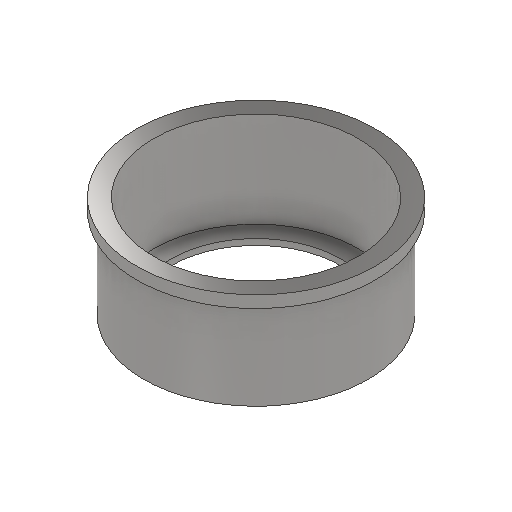
# Autodesk Inventor part: B_pipe_flange_spacer_5
Saved by Autodesk Inventor 2026.2 (Build 302298000, 298)
## iProperties
Created: 2026-07-10
Part Number: B_pipe_flange_spacer_5
Material: ステンレス鋼
Document SubType Name: Modeling
Designer: zetsu
Density: 8 g/cm^3
Appearance: 半つや出し
Author: zetsu
Autodesk Inventor part; units mm, degrees
ref_plane "YZ Plane" through (0, 0, 0) normal (1, 0, 0) x (0, 1, 0)
ref_plane "XZ Plane" through (0, 0, 0) normal (0, 1, 0) x (-1, 0, 0)
ref_plane "XY Plane" through (0, 0, 0) normal (0, 0, 1) x (1, 0, 0)
sketch "スケッチ1" plane through (0, 0, 0) normal (0, 1, 0) x (-1, 0, 0)
  circle A0 centre (0, 0) radius 18.85
  circle A1 centre (0, 0) radius 14.2
  dimension "d0" = 37.7
  dimension "d1" = 28.4
  constraints: 2 centre point, 2 coincident
  measures "d0" diameter of A0
  measures "d1" diameter of A1
extrude "押し出し1" add sketch "スケッチ1" along normal blind 15
sketch "スケッチ2" plane through (0, 15, 0) normal (0, 1, 0) x (1, 0, 0)
  circle A0 centre (0, 0) radius 17.15
  dimension "d4" = 34.3
  constraints: 1 centre point, 1 coincident
  measures "d4" diameter of A0
extrude "押し出し2" cut sketch "スケッチ2" against normal blind 14
sketch "スケッチ3" plane through (0, 15, 0) normal (0, 1, 0) x (1, 0, 0)
  circle A0 centre (0, 0) radius 17.15
  circle A1 centre (0, 0) radius 20
  dimension "d7" = 34.3
  dimension "d8" = 40
  constraints: 2 centre point, 2 coincident
  measures "d7" diameter of A0
  measures "d8" diameter of A1
extrude "押し出し3" add sketch "スケッチ3" along normal blind 2
